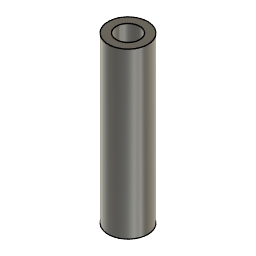
PivotPin (Autodesk Fusion 360 design; units mm, degrees)
part number: 2026-05-26-23-25-24-606
Autodesk Fusion 360 part; units mm, degrees
sketch "TopView" plane through (0, 0, 0) normal (0, 0, 1) x (1, 0, 0)
  circle A0 centre (0, 0) radius 7.8
  circle A1 centre (0, 0) radius 4.6
  dimension "d1" = 15.6
  dimension "d2" = 9.2
  constraint coincident A0.centre A1.centre
  constraint concentric A0 A1
  measures "d1" diameter of A0
  measures "d2" diameter of A1
extrude "Extrude1" add sketch "TopView" along normal blind 64.8
named bodies: "PivotPin"
